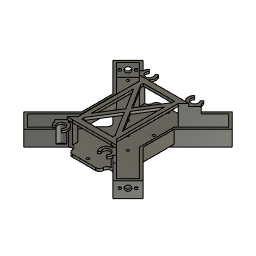
Frame_UAV2024 v2 (Autodesk Fusion 360 design; units mm, degrees)
Autodesk Fusion 360 part; units mm, degrees
sketch "スケッチ1" plane through (0, 0, 0) normal (0, 0, 1) x (1, 0, 0)
  line L0 (12, 34) -> (-12, 34)
  line L1 (-12, 34) -> (-12, -34)
  line L2 (-12, -34) -> (12, -34)
  line L3 (12, -34) -> (12, 34)
  line L4 (12, 34) -> (-12, -34) construction
  line L5 (-12, 34) -> (12, -34) construction
  line L6 (0, 0) -> (38.890873, 38.890873)
  line L7 (34.471456, 43.31029) -> (43.31029, 34.471456)
  line L8 (34.471456, 43.31029) -> (43.31029, 34.471456)
  line L9 (43.31029, 34.471456) -> (21.955666, 13.116831)
  line L10 (21.955666, 13.116831) -> (13.116831, 21.955666)
  line L11 (13.116831, 21.955666) -> (34.471456, 43.31029)
  line L12 (-34.471456, 43.31029) -> (-13.116831, 21.955666)
  line L13 (-13.116831, 21.955666) -> (-21.955666, 13.116831)
  line L14 (-21.955666, 13.116831) -> (-43.31029, 34.471456)
  line L15 (-43.31029, 34.471456) -> (-34.471456, 43.31029)
  line L16 (-43.31029, -34.471456) -> (-21.955666, -13.116831)
  line L17 (-21.955666, -13.116831) -> (-13.116831, -21.955666)
  line L18 (-13.116831, -21.955666) -> (-34.471456, -43.31029)
  line L19 (-34.471456, -43.31029) -> (-43.31029, -34.471456)
  line L20 (34.471456, -43.31029) -> (13.116831, -21.955666)
  line L21 (13.116831, -21.955666) -> (21.955666, -13.116831)
  line L22 (21.955666, -13.116831) -> (43.31029, -34.471456)
  line L23 (43.31029, -34.471456) -> (34.471456, -43.31029)
  line L24 (-10.288404, 21.955666) -> (-21.955666, 10.288404)
  line L25 (-21.955666, 10.288404) -> (-46.138717, 34.471456)
  line L26 (-46.138717, 34.471456) -> (-34.471456, 46.138717)
  line L27 (-34.471456, 46.138717) -> (-10.288404, 21.955666)
  line L28 (46.138717, 34.471456) -> (21.955666, 10.288404)
  line L29 (21.955666, 10.288404) -> (10.288404, 21.955666)
  line L30 (10.288404, 21.955666) -> (34.471456, 46.138717)
  line L31 (34.471456, 46.138717) -> (46.138717, 34.471456)
  line L32 (-46.138717, -34.471456) -> (-21.955666, -10.288404)
  line L33 (-21.955666, -10.288404) -> (-10.288404, -21.955666)
  line L34 (-10.288404, -21.955666) -> (-34.471456, -46.138717)
  line L35 (-34.471456, -46.138717) -> (-46.138717, -34.471456)
  line L36 (21.955666, -10.288404) -> (46.138717, -34.471456)
  line L37 (46.138717, -34.471456) -> (34.471456, -46.138717)
  line L38 (34.471456, -46.138717) -> (10.288404, -21.955666)
  line L39 (10.288404, -21.955666) -> (21.955666, -10.288404)
  line L40 (-10.288404, 21.955666) -> (-12, 23.667262)
  line L41 (10.288404, 21.955666) -> (12, 23.667262)
  line L42 (-10.288404, -21.955666) -> (-12, -23.667262)
  line L43 (10.288404, -21.955666) -> (12, -23.667262)
  line L44 (-21.955666, 10.288404) -> (-12, 0.332738)
  line L45 (-21.955666, 10.288404) -> (-6.411762, 10.288404) construction
  line L46 (-21.955666, -10.288404) -> (-12, -0.332738)
  line L47 (21.955666, 10.288404) -> (12, 0.332738)
  line L48 (21.955666, -10.288404) -> (12, -0.332738)
  dimension "d1" = 24
  dimension "d2" = 68
  dimension "d8" = 55
  dimension "d9" = 12.5
  dimension "d10" = 30.2
  dimension "d14" = 360
  dimension "d15" = -2
  dimension "d16" = -2
  dimension "d17" = -2
  dimension "d18" = -2
  dimension "d101" = 45
  dimension "d102" = 90
  dimension "d103" = 90
  constraint horizontal L0
  constraint perpendicular L0 L1
  constraint parallel L0 L2
  constraint parallel L1 L3
  constraint coincident L4 L6.start
  constraint coincident L5 L6.start
  constraint coincident L6.start origin
  constraint perpendicular L6 L7
  constraint perpendicular L8 L9
  constraint parallel L8 L10
  constraint parallel L9 L11
  constraint perpendicular L24 L40
  constraint perpendicular L29 L41
  constraint perpendicular L33 L42
  constraint perpendicular L39 L43
  constraint horizontal L45
  constraint perpendicular L24 L44
  constraint perpendicular L29 L47
  measures "d1" distance of L1.end L2.end
  measures "d2" distance of L0.end L1.end
  measures "d101" angle of L44 L45
  measures "d102" angle of L44 L46
  measures "d103" angle of L47 L48
extrude "押し出し1" add sketch "スケッチ1" along normal blind 2 contours L0 L1 L2 L3 L24 L27 L29 L30 L33 L34 L38 L39 L40 L41 L42 L43 | L3 L28 L29 L30 L31 | L3 L29 L30 L41 | L1 L24 L27 L40 | L1 L24 L25 L26 L27 | L3 L6 L29 | L1 L24 L44 | L3 L6 L29 L47 | L1 L33 L46 | L3 L39 L48 | L1 L33 L34 L42 | L1 L32 L33 L34 L35 | L3 L36 L37 L38 L39 | L3 L38 L39 L43 | L6 L7 L8 L10 L11 | L6 L7 L8 L9 L10 | L12 L13 L14 L15 | L16 L17 L18 L19 | L20 L21 L22 L23 picked at (3.429468, -7.540381) picked at (37.134891, 26.410438) picked at (11.429468, 21.955666) picked at (-11.429468, 21.955666) picked at (-30.016683, 19.29223) picked at (13.374012, 16.122035) picked at (-15.318555, 10.288404) picked at (15.318555, 7.540381) picked at (-15.318555, -10.288404) picked at (15.318555, -10.288404) picked at (-11.429468, -21.955666) picked at (-30.016683, -19.29223) picked at (30.016683, -19.29223) picked at (11.429468, -21.955666) picked at (28.826386, 34.718943) picked at (27.600735, 21.708178) picked at (-23.181317, 26.127596) picked at (-26.127596, -23.181317) picked at (23.181317, -26.127596)
sketch "スケッチ2" plane through (0, 0, 2) normal (0, 0, 1) x (-1, 0, 0)
  line L0 (12, 0.332738) -> (46.138717, 34.471456)
  line L1 (46.138717, 34.471456) -> (34.471456, 46.138717)
  line L2 (34.471456, 46.138717) -> (12, 23.667262)
  line L3 (12, 23.667262) -> (12, 34)
  line L4 (12, 34) -> (-12, 34)
  line L5 (-12, 34) -> (-12, 23.667262)
  line L6 (-12, 23.667262) -> (-34.471456, 46.138717)
  line L7 (-34.471456, 46.138717) -> (-46.138717, 34.471456)
  line L8 (-46.138717, 34.471456) -> (-12, 0.332738)
  line L9 (-12, 0.332738) -> (-12, -0.332738)
  line L10 (-12, -0.332738) -> (-46.138717, -34.471456)
  line L11 (-46.138717, -34.471456) -> (-34.471456, -46.138717)
  line L12 (-34.471456, -46.138717) -> (-12, -23.667262)
  line L13 (-12, -23.667262) -> (-12, -34)
  line L14 (-12, -34) -> (12, -34)
  line L15 (12, -34) -> (12, -23.667262)
  line L16 (12, -23.667262) -> (34.471456, -46.138717)
  line L17 (34.471456, -46.138717) -> (46.138717, -34.471456)
  line L18 (46.138717, -34.471456) -> (12, -0.332738)
  line L19 (12, -0.332738) -> (12, 0.332738)
  line L20 (-46.138717, -34.471456) -> (-34.471456, -46.138717)
  line L21 (-34.471456, -46.138717) -> (-12, -23.667262)
  line L22 (-12, -23.667262) -> (-23.667262, -12)
  line L23 (-23.667262, -12) -> (-46.138717, -34.471456)
  line L24 (-14.828427, -23.667262) -> (-23.667262, -14.828427)
  line L25 (-23.667262, -14.828427) -> (-43.31029, -34.471456)
  line L26 (-43.31029, -34.471456) -> (-34.471456, -43.31029)
  line L27 (-34.471456, -43.31029) -> (-14.828427, -23.667262)
  line L28 (-14.828427, -23.667262) -> (-13.414214, -22.253048)
  line L29 (-23.667262, -14.828427) -> (-22.253048, -13.414214)
  line L30 (-12, -23.667262) -> (-13.414214, -22.253048)
  line L31 (-22.253048, -13.414214) -> (-23.667262, -12)
  line L32 (43.31029, -34.471456) -> (23.667262, -14.828427)
  line L33 (34.471456, -43.31029) -> (43.31029, -34.471456)
  line L34 (14.828427, -23.667262) -> (34.471456, -43.31029)
  line L35 (14.828427, -23.667262) -> (13.414214, -22.253048)
  line L36 (23.667262, -14.828427) -> (22.253048, -13.414214)
  line L37 (23.667262, -12) -> (22.253048, -13.414214)
  line L38 (13.414214, -22.253048) -> (12, -23.667262)
  line L39 (34.471456, 43.31029) -> (14.828427, 23.667262)
  line L40 (43.31029, 34.471456) -> (34.471456, 43.31029)
  line L41 (23.667262, 14.828427) -> (43.31029, 34.471456)
  line L42 (23.667262, 14.828427) -> (22.253048, 13.414214)
  line L43 (14.828427, 23.667262) -> (13.414214, 22.253048)
  line L44 (12, 23.667262) -> (13.414214, 22.253048)
  line L45 (22.253048, 13.414214) -> (23.667262, 12)
  line L46 (-43.31029, 34.471456) -> (-23.667262, 14.828427)
  line L47 (-34.471456, 43.31029) -> (-43.31029, 34.471456)
  line L48 (-14.828427, 23.667262) -> (-34.471456, 43.31029)
  line L49 (-14.828427, 23.667262) -> (-13.414214, 22.253048)
  line L50 (-23.667262, 14.828427) -> (-22.253048, 13.414214)
  line L51 (-23.667262, 12) -> (-22.253048, 13.414214)
  line L52 (-13.414214, 22.253048) -> (-12, 23.667262)
  dimension "d105" = -2
  dimension "d107" = 360
  constraint perpendicular L20 L21
  constraint parallel L20 L22
  constraint parallel L21 L23
  constraint perpendicular L12 L20
  constraint perpendicular L22 L28
  constraint perpendicular L22 L29
  constraint perpendicular L28 L30
extrude "押し出し2" add sketch "スケッチ2" along normal blind 10 contours L0 L1 L2 L39 L40 L41 L42 L43 L44 L45 | L16 L17 L18 L32 L33 L34 L35 L36 L37 L38 | L6 L7 L8 L46 L47 L48 L49 L50 L51 L52 | L10 L11 L12 L20 L21 L22 L23 L25 L26 L27 L28 L29 L30 L31 picked at (31.157747, 20.433294) picked at (20.433294, -31.157747) picked at (-20.433294, 31.157747) picked at (-31.157747, -20.433294)
sketch "スケッチ3" plane through (-40.305087, 40.305087, 0) normal (-0.707107, 0.707107, 0) x (-0.707107, -0.707107, 0)
  line L0 (-8.25, 0) -> (8.25, 0)
  line L1 (8.25, 0) -> (8.25, 12)
  line L2 (8.25, 12) -> (-8.25, 12)
  line L3 (-8.25, 12) -> (-8.25, 0)
  line L4 (0, 12) -> (0, 7)
  circle A0 centre (0, 7) radius 2.1
  line L5 (0, 7) -> (4.5, 7)
  circle A1 centre (4.5, 7) radius 1
  line L6 (0, 7) -> (-4.5, 7)
  circle A2 centre (-4.5, 7) radius 1
  dimension "d33" = 4.2
  dimension "d34" = 4.5
  dimension "d35" = 2
  dimension "d36" = 4.5
  dimension "d37" = 2
  constraint midpoint L2 L4.start
  constraint perpendicular L2 L4
  constraint coincident L4.end A0.centre
  constraint perpendicular L4 L5
  constraint coincident L5.end A1.centre
  constraint perpendicular L4 L6
  constraint coincident L6.end A2.centre
  measures "d33" diameter of A0
  measures "d34" distance of L4.end L5.end
  measures "d35" diameter of A1
  measures "d36" distance of L4.end L6.end
  measures "d37" diameter of A2
extrude "押し出し3" cut sketch "スケッチ3" against normal blind 2 contours L4 A0 L5 | L4 A0 L6 | A0 L5 L6 | A1 | A2 picked at (1.308387, 7.488003) picked at (-1.117902, 7.836851) picked at (-1.392182, 6.895671) picked at (4.70783, 6.807162) picked at (-4.121993, 6.641138)
pattern_circular "C パターン1" count 4 over 360 about axis through (0, 0, 1.75) along (0, 0, 1) of "押し出し3"
ref_plane "作業平面4" through (0, 0, 12) normal (0, 0, 1) x (1, 0, 0)
sketch "スケッチ24" plane through (0, 0, 12) normal (0, 0, 1) x (1, 0, 0)
  line L0 (17.5, 34) -> (-17.5, 34)
  line L1 (-17.5, 34) -> (-17.5, -34)
  line L2 (-17.5, -34) -> (17.5, -34)
  line L3 (17.5, -34) -> (17.5, 34)
  line L4 (17.5, 34) -> (-17.5, -34) construction
  line L5 (-17.5, 34) -> (17.5, -34) construction
  circle A0 centre (-17.5, 34) radius 3
  line L6 (-46.138717, -34.471456) -> (-12, -0.332738)
  line L7 (-12, -0.332738) -> (-12, 0.332738)
  line L8 (-12, 0.332738) -> (-46.138717, 34.471456)
  line L9 (-46.138717, 34.471456) -> (-34.471456, 46.138717)
  line L10 (-34.471456, 46.138717) -> (-12, 23.667262)
  line L11 (-12, 23.667262) -> (-12, 34)
  line L12 (-12, 34) -> (12, 34)
  line L13 (12, 34) -> (12, 23.667262)
  line L14 (12, 23.667262) -> (34.471456, 46.138717)
  line L15 (34.471456, 46.138717) -> (46.138717, 34.471456)
  line L16 (46.138717, 34.471456) -> (12, 0.332738)
  line L17 (12, 0.332738) -> (12, -0.332738)
  line L18 (12, -0.332738) -> (46.138717, -34.471456)
  line L19 (46.138717, -34.471456) -> (34.471456, -46.138717)
  line L20 (34.471456, -46.138717) -> (12, -23.667262)
  line L21 (12, -23.667262) -> (12, -34)
  line L22 (12, -34) -> (-12, -34)
  line L23 (-12, -34) -> (-12, -23.667262)
  line L24 (-12, -23.667262) -> (-34.471456, -46.138717)
  line L25 (-34.471456, -46.138717) -> (-46.138717, -34.471456)
  circle A1 centre (17.5, 34) radius 3
  circle A2 centre (-17.5, -34) radius 3
  circle A3 centre (17.5, -34) radius 3
  circle A4 centre (-17.5, 34) radius 5
  circle A5 centre (17.5, 34) radius 5
  circle A6 centre (-17.5, -34) radius 5
  circle A7 centre (17.5, -34) radius 5
  dimension "d119" = 35
  dimension "d120" = 68
  dimension "d122" = 6
  dimension "d125" = 6
  dimension "d126" = 6
  dimension "d127" = 6
  dimension "d152" = 10
  dimension "d153" = 10
  dimension "d154" = 10
  dimension "d155" = 10
  constraint horizontal L0
  constraint perpendicular L0 L1
  constraint parallel L0 L2
  constraint parallel L1 L3
  constraint coincident L4 origin
  constraint coincident L5 origin
  constraint coincident L0.end L1.start
  constraint coincident L0.start L3.end
  constraint coincident L1.end L2.start
  constraint coincident L2.end L3.start
  constraint concentric A0 A4
  constraint concentric A1 A5
  constraint concentric A2 A6
  constraint concentric A3 A7
  measures "d119" distance of L1.end L2.end
  measures "d120" distance of L0.end L1.end
  measures "d122" diameter of A0
  measures "d125" diameter of A1
  measures "d126" diameter of A2
  measures "d127" diameter of A3
  measures "d152" diameter of A4
  measures "d153" diameter of A5
  measures "d154" diameter of A6
  measures "d155" diameter of A7
extrude "押し出し22" add sketch "スケッチ24" against normal blind 1.5 contours L0 L3 L14 A1 A5 | L0 L3 L14 A1 A5 | L0 L1 A0 L10 A4 | L0 L1 A0 L10 A4 | L2 L3 L20 A3 A7 | L2 L3 L20 A3 A7 | L1 L2 L24 A2 A6 | L1 L2 L24 A2 A6 picked at (21.79405, 34.503832) picked at (17.071241, 29.757399) picked at (-17.071241, 29.757399) picked at (-21.804015, 34.403857) picked at (21.79405, -34.503832) picked at (17.071241, -29.757399) picked at (-17.071241, -29.757399) picked at (-21.804015, -34.403857)
sketch "スケッチ25" plane through (0, 0, 2) normal (0, 0, 1) x (-1, 0, 0)
  line L0 (22.253048, -13.414214) -> (23.667262, -12)
  line L1 (23.667262, -12) -> (12, -0.332738)
  line L2 (12, -0.332738) -> (12, 0.332738)
  line L3 (12, 0.332738) -> (23.667262, 12)
  line L4 (23.667262, 12) -> (22.253048, 13.414214)
  line L5 (22.253048, 13.414214) -> (43.31029, 34.471456)
  line L6 (43.31029, 34.471456) -> (34.471456, 43.31029)
  line L7 (34.471456, 43.31029) -> (13.414214, 22.253048)
  line L8 (13.414214, 22.253048) -> (12, 23.667262)
  line L9 (12, 23.667262) -> (12, 34)
  line L10 (12, 34) -> (-12, 34)
  line L11 (-12, 34) -> (-12, 23.667262)
  line L12 (-12, 23.667262) -> (-13.414214, 22.253048)
  line L13 (-13.414214, 22.253048) -> (-34.471456, 43.31029)
  line L14 (-34.471456, 43.31029) -> (-43.31029, 34.471456)
  line L15 (-43.31029, 34.471456) -> (-22.253048, 13.414214)
  line L16 (-22.253048, 13.414214) -> (-23.667262, 12)
  line L17 (-23.667262, 12) -> (-12, 0.332738)
  line L18 (-12, 0.332738) -> (-12, -0.332738)
  line L19 (-12, -0.332738) -> (-23.667262, -12)
  line L20 (-23.667262, -12) -> (-22.253048, -13.414214)
  line L21 (-22.253048, -13.414214) -> (-43.31029, -34.471456)
  line L22 (-43.31029, -34.471456) -> (-34.471456, -43.31029)
  line L23 (-34.471456, -43.31029) -> (-13.414214, -22.253048)
  line L24 (-13.414214, -22.253048) -> (-12, -23.667262)
  line L25 (-12, -23.667262) -> (-12, -34)
  line L26 (-12, -34) -> (12, -34)
  line L27 (12, -34) -> (12, -23.667262)
  line L28 (12, -23.667262) -> (13.414214, -22.253048)
  line L29 (13.414214, -22.253048) -> (34.471456, -43.31029)
  line L30 (34.471456, -43.31029) -> (43.31029, -34.471456)
  line L31 (43.31029, -34.471456) -> (22.253048, -13.414214)
  line L32 (17.5, -34) -> (-17.5, -34)
  line L33 (-17.5, -34) -> (-17.5, 34)
  line L34 (-17.5, 34) -> (17.5, 34)
  line L35 (17.5, 34) -> (17.5, -34)
  line L36 (17.5, -34) -> (-17.5, 34) construction
  line L37 (-17.5, -34) -> (17.5, 34) construction
  circle A0 centre (17.5, -34) radius 4.5
  circle A1 centre (-17.5, -34) radius 4.5
  circle A2 centre (17.5, 34) radius 4.5
  circle A3 centre (-17.5, 34) radius 4.5
  dimension "d130" = 35
  dimension "d131" = 68
  dimension "d132" = 9
  dimension "d133" = 9
  dimension "d134" = 9
  dimension "d135" = 9
  constraint horizontal L32
  constraint perpendicular L32 L33
  constraint parallel L32 L34
  constraint parallel L33 L35
  constraint coincident L36 origin
  constraint coincident L37 origin
  constraint coincident L32.start L35.end
  constraint coincident L32.end L33.start
  constraint coincident L34.end L35.start
  constraint coincident L33.end L34.start
  measures "d130" distance of L33.end L34.end
  measures "d131" distance of L32.end L33.end
  measures "d132" diameter of A0
  measures "d133" diameter of A1
  measures "d134" diameter of A2
  measures "d135" diameter of A3
extrude "押し出し23" cut sketch "スケッチ25" along normal blind 8.5 contours L32 L35 A0 | L32 L35 A0 | L34 L35 A2 | L34 L35 A2 | L32 L33 A1 | L32 L33 A1 | L33 L34 A3 | L33 L34 A3 picked at (14.516754, -34.223563) picked at (14.873672, -32.565916) picked at (14.515268, 33.786528) picked at (14.583395, 34.665696) picked at (-14.580825, -34.655523) picked at (-14.576028, -33.363929) picked at (-14.515268, 33.786528) picked at (-18.57676, 31.208606)
sketch "スケッチ26" plane through (0, 0, 12) normal (0, 0, 1) x (1, 0, 0)
  circle A0 centre (-17.5, 34) radius 3
  circle A1 centre (17.5, 34) radius 3
  circle A2 centre (-17.5, -34) radius 3
  circle A3 centre (17.5, -34) radius 3
  line L0 (-17.5, 34) -> (-13.610913, 37.889087)
  line L1 (-17.5, 34) -> (-12, 34) construction
  arc A4 (-13.610913, 37.889087) -> (-21.389087, 37.889087) centre (-17.5, 34) ccw
  line L2 (-17.5, 34) -> (-21.389087, 37.889087)
  line L3 (0, 2.5) -> (0, 20)
  line L4 (17.5, 34) -> (21.389087, 37.889087)
  line L5 (17.5, 34) -> (13.610913, 37.889087)
  arc A5 (21.389087, 37.889087) -> (13.610913, 37.889087) centre (17.5, 34) ccw
  line L6 (20, 0) -> (2.5, 0)
  line L7 (-17.5, -34) -> (-13.610913, -37.889087)
  line L8 (-17.5, -34) -> (-21.389087, -37.889087)
  arc A6 (-21.389087, -37.889087) -> (-13.610913, -37.889087) centre (-17.5, -34) ccw
  line L9 (17.5, -34) -> (21.389087, -37.889087)
  line L10 (17.5, -34) -> (13.610913, -37.889087)
  arc A7 (13.610913, -37.889087) -> (21.389087, -37.889087) centre (17.5, -34) ccw
  dimension "d138" = 45
  constraint horizontal L1
  constraint coincident A0.centre L0.start
  constraint symmetric A0.centre L3 A1.centre
  constraint symmetric A4 L3 A5
  constraint symmetric A0.centre L6 A2.centre
  constraint symmetric A4 L6 A6
  constraint symmetric A1.centre L6 A3.centre
  constraint symmetric A5 L6 A7
  measures "d138" angle of L0 L1
extrude "押し出し24" cut sketch "スケッチ26" against normal blind 1.5 contours A0 L0 A4 L2 | A1 L4 L5 A5 | A2 L7 L8 A6 | A3 L9 L10 A7 picked at (-15.043452, 37.954416) picked at (19.956548, 37.954416) picked at (-15.043452, -37.954416) picked at (19.368772, -38.263769)
sketch "スケッチ27" plane through (0, 0, 0) normal (0, 0, -1) x (1, 0, 0)
  line L0 (-46.138717, 34.471456) -> (-12, 0.332738)
  line L1 (-12, 0.332738) -> (-12, -0.332738)
  line L2 (-12, -0.332738) -> (-46.138717, -34.471456)
  line L3 (-46.138717, -34.471456) -> (-34.471456, -46.138717)
  line L4 (-34.471456, -46.138717) -> (-12, -23.667262)
  line L5 (-12, -23.667262) -> (-12, -34)
  line L6 (-12, -34) -> (12, -34)
  line L7 (12, -34) -> (12, -23.667262)
  line L8 (12, -23.667262) -> (34.471456, -46.138717)
  line L9 (34.471456, -46.138717) -> (46.138717, -34.471456)
  line L10 (46.138717, -34.471456) -> (12, -0.332738)
  line L11 (12, -0.332738) -> (12, 0.332738)
  line L12 (12, 0.332738) -> (46.138717, 34.471456)
  line L13 (46.138717, 34.471456) -> (34.471456, 46.138717)
  line L14 (34.471456, 46.138717) -> (12, 23.667262)
  line L15 (12, 23.667262) -> (12, 34)
  line L16 (12, 34) -> (-12, 34)
  line L17 (-12, 34) -> (-12, 23.667262)
  line L18 (-12, 23.667262) -> (-34.471456, 46.138717)
  line L19 (-34.471456, 46.138717) -> (-46.138717, 34.471456)
  line L20 (10, -10) -> (-10, -10)
  line L21 (-10, -10) -> (-10, 10)
  line L22 (-10, 10) -> (10, 10)
  line L23 (10, 10) -> (10, -10)
  line L24 (10, -10) -> (-10, 10) construction
  line L25 (-10, -10) -> (10, 10) construction
  circle A0 centre (-10, 10) radius 0.9
  circle A1 centre (-10, 10) radius 2.5
  circle A2 centre (-10, -10) radius 2.5
  circle A3 centre (-10, -10) radius 0.9
  circle A4 centre (10, -10) radius 2.5
  circle A5 centre (10, -10) radius 0.9
  circle A6 centre (10, 10) radius 2.5
  circle A7 centre (10, 10) radius 0.9
  dimension "d141" = 20
  dimension "d142" = 20
  dimension "d143" = 1.8
  dimension "d144" = 5
  dimension "d146" = 360
  constraint horizontal L20
  constraint perpendicular L20 L21
  constraint parallel L20 L22
  constraint parallel L21 L23
  constraint coincident L24 origin
  constraint coincident L25 origin
  constraint coincident L21.end L22.start
  measures "d141" distance of L21.end L22.end
  measures "d142" distance of L20.end L21.end
  measures "d143" diameter of A0
  measures "d144" diameter of A1
extrude "押し出し25" add sketch "スケッチ27" along normal blind 5 contours L20 L21 A2 A3 | L20 L21 A2 A3 | L20 L23 A4 A5 | L20 L23 A4 A5 | L21 L22 A0 A1 | L21 L22 A0 A1 | L22 L23 A6 A7 | L22 L23 A6 A7 picked at (-9.929804, -11.960206) picked at (-8.628033, -8.597767) picked at (8.044869, -9.83871) picked at (11.957359, -10.124202) picked at (-10.122275, 8.042353) picked at (-9.881404, 8.041815) picked at (8.078625, 9.603933) picked at (8.045992, 10.168915)
sketch "スケッチ28" plane through (0, 0, 12) normal (0, 0, 1) x (1, 0, 0)
  line L0 (-12, 34.000001) -> (12, 34.000001)
  line L1 (12, 34.000001) -> (12, -34.000001)
  line L2 (12, -34.000001) -> (-12, -34.000001)
  line L3 (-12, -34.000001) -> (-12, 34.000001)
  line L4 (-12, 34.000001) -> (12, -34.000001) construction
  line L5 (12, 34.000001) -> (-12, -34.000001) construction
  line L6 (15, 37.000001) -> (15, -37.000001)
  line L7 (15, -37.000001) -> (-15, -37.000001)
  line L8 (-15, -37.000001) -> (-15, 37.000001)
  line L9 (-15, 37.000001) -> (15, 37.000001)
  line L10 (-13.964466, 37.535534) -> (-15.37868, 36.12132)
  arc A0 (-15.37868, 36.12132) -> (-19.62132, 36.12132) centre (-17.5, 34) cw
  line L11 (-19.62132, 36.12132) -> (-21.035534, 37.535534)
  arc A1 (-21.035534, 37.535534) -> (-22.497291, 34.164553) centre (-17.5, 34) ccw
  line L12 (-22.497291, 34.164553) -> (-34.471456, 46.138717)
  line L13 (-34.471456, 46.138717) -> (-46.138717, 34.471456)
  line L14 (-46.138717, 34.471456) -> (-23.667262, 12)
  line L15 (-23.667262, 12) -> (-22.253048, 13.414214)
  line L16 (-22.253048, 13.414214) -> (-43.31029, 34.471456)
  line L17 (-43.31029, 34.471456) -> (-34.471456, 43.31029)
  line L18 (-34.471456, 43.31029) -> (-13.414214, 22.253048)
  line L19 (-13.414214, 22.253048) -> (-12, 23.667262)
  line L20 (-12, 23.667262) -> (-17.335447, 29.002709)
  arc A2 (-17.335447, 29.002709) -> (-13.964466, 37.535534) centre (-17.5, 34) ccw
  line L21 (21.035534, 37.535534) -> (19.62132, 36.12132)
  arc A3 (19.62132, 36.12132) -> (15.37868, 36.12132) centre (17.5, 34) cw
  line L22 (15.37868, 36.12132) -> (13.964466, 37.535534)
  arc A4 (13.964466, 37.535534) -> (17.335447, 29.002709) centre (17.5, 34) ccw
  line L23 (17.335447, 29.002709) -> (12, 23.667262)
  line L24 (12, 23.667262) -> (13.414214, 22.253048)
  line L25 (13.414214, 22.253048) -> (34.471456, 43.31029)
  line L26 (34.471456, 43.31029) -> (43.31029, 34.471456)
  line L27 (43.31029, 34.471456) -> (22.253048, 13.414214)
  line L28 (22.253048, 13.414214) -> (23.667262, 12)
  line L29 (23.667262, 12) -> (46.138717, 34.471456)
  line L30 (46.138717, 34.471456) -> (34.471456, 46.138717)
  line L31 (34.471456, 46.138717) -> (22.497291, 34.164553)
  arc A5 (22.497291, 34.164553) -> (21.035534, 37.535534) centre (17.5, 34) ccw
  line L32 (-21.035534, -37.535534) -> (-19.62132, -36.12132)
  arc A6 (-19.62132, -36.12132) -> (-15.37868, -36.12132) centre (-17.5, -34) cw
  line L33 (-15.37868, -36.12132) -> (-13.964466, -37.535534)
  arc A7 (-13.964466, -37.535534) -> (-17.335447, -29.002709) centre (-17.5, -34) ccw
  line L34 (-17.335447, -29.002709) -> (-12, -23.667262)
  line L35 (-12, -23.667262) -> (-13.414214, -22.253048)
  line L36 (-13.414214, -22.253048) -> (-34.471456, -43.31029)
  line L37 (-34.471456, -43.31029) -> (-43.31029, -34.471456)
  line L38 (-43.31029, -34.471456) -> (-22.253048, -13.414214)
  line L39 (-22.253048, -13.414214) -> (-23.667262, -12)
  line L40 (-23.667262, -12) -> (-46.138717, -34.471456)
  line L41 (-46.138717, -34.471456) -> (-34.471456, -46.138717)
  line L42 (-34.471456, -46.138717) -> (-22.497291, -34.164553)
  arc A8 (-22.497291, -34.164553) -> (-21.035534, -37.535534) centre (-17.5, -34) ccw
  line L43 (13.964466, -37.535534) -> (15.37868, -36.12132)
  arc A9 (15.37868, -36.12132) -> (19.62132, -36.12132) centre (17.5, -34) cw
  line L44 (19.62132, -36.12132) -> (21.035534, -37.535534)
  arc A10 (21.035534, -37.535534) -> (22.497291, -34.164553) centre (17.5, -34) ccw
  line L45 (22.497291, -34.164553) -> (34.471456, -46.138717)
  line L46 (34.471456, -46.138717) -> (46.138717, -34.471456)
  line L47 (46.138717, -34.471456) -> (23.667262, -12)
  line L48 (23.667262, -12) -> (22.253048, -13.414214)
  line L49 (22.253048, -13.414214) -> (43.31029, -34.471456)
  line L50 (43.31029, -34.471456) -> (34.471456, -43.31029)
  line L51 (34.471456, -43.31029) -> (13.414214, -22.253048)
  line L52 (13.414214, -22.253048) -> (12, -23.667262)
  line L53 (12, -23.667262) -> (17.335447, -29.002709)
  arc A11 (17.335447, -29.002709) -> (13.964466, -37.535534) centre (17.5, -34) ccw
  dimension "d149" = -3
  constraint horizontal L0
  constraint perpendicular L0 L1
  constraint parallel L0 L2
  constraint parallel L1 L3
  constraint coincident L4 origin
  constraint coincident L5 origin
extrude "押し出し26" cut sketch "スケッチ28" against normal blind 10 contours L8 L18 L19 L20 | L6 L23 L24 L25 | L8 L34 L35 L36 | L6 L51 L52 L53 picked at (-14, 24.724453) picked at (14, 24.724453) picked at (-14, -24.724453) picked at (14, -24.724453)
extrude "押し出し27" cut 4 faces at (9.731307, 10.009657, 0) (-10.083244, 10.032671, 0) (-10.182869, -9.709695, 0) (10.356587, -10.144182, 0) along direction (0, 0, 1) blind 2
fillet "フィレット1" radius 3 8 edges at (12, 23.667262, 1) (-12, 23.667262, 1) (12, -23.667262, 1) (-12, -23.667262, 1) (-12, 0.332738, 1) (-12, -0.332738, 1) (12, -0.332738, 1) (12, 0.332738, 1)
fillet "フィレット2" radius 3 4 edges at (12, 34, 1) (-12, 34, 1) (-12, -34, 1) (12, -34, 1)
sketch "スケッチ29" plane through (0, 0, 2) normal (0, 0, 1) x (-1, 0, 0)
  arc A0 (-9, 34) -> (-12, 31) centre (-9, 31) ccw
  line L0 (-12, 31) -> (-12, 30.909903)
  arc A1 (-15, 27.909903) -> (-12, 30.909903) centre (-15, 30.909903) ccw
  line L1 (-15, 27.909903) -> (-15, 23.838835)
  line L2 (-15, 23.838835) -> (-34.471456, 43.31029)
  line L3 (-34.471456, 43.31029) -> (-43.31029, 34.471456)
  line L4 (-43.31029, 34.471456) -> (-22.253048, 13.414214)
  line L5 (-22.253048, 13.414214) -> (-23.667262, 12)
  line L6 (-23.667262, 12) -> (-13.788582, 2.12132)
  arc A2 (-13.788582, -2.12132) -> (-13.788582, 2.12132) centre (-15.909903, 0) ccw
  line L7 (-13.788582, -2.12132) -> (-23.667262, -12)
  line L8 (-23.667262, -12) -> (-22.253048, -13.414214)
  line L9 (-22.253048, -13.414214) -> (-43.31029, -34.471456)
  line L10 (-43.31029, -34.471456) -> (-34.471456, -43.31029)
  line L11 (-34.471456, -43.31029) -> (-15, -23.838835)
  line L12 (-15, -23.838835) -> (-15, -27.909903)
  arc A3 (-12, -30.909903) -> (-15, -27.909903) centre (-15, -30.909903) ccw
  line L13 (-12, -30.909903) -> (-12, -31)
  arc A4 (-12, -31) -> (-9, -34) centre (-9, -31) ccw
  line L14 (-9, -34) -> (9, -34)
  arc A5 (9, -34) -> (12, -31) centre (9, -31) ccw
  line L15 (12, -31) -> (12, -30.909903)
  arc A6 (15, -27.909903) -> (12, -30.909903) centre (15, -30.909903) ccw
  line L16 (15, -27.909903) -> (15, -23.838835)
  line L17 (15, -23.838835) -> (34.471456, -43.31029)
  line L18 (34.471456, -43.31029) -> (43.31029, -34.471456)
  line L19 (43.31029, -34.471456) -> (22.253048, -13.414214)
  line L20 (22.253048, -13.414214) -> (23.667262, -12)
  line L21 (23.667262, -12) -> (13.788582, -2.12132)
  line L22 (13.788582, 2.12132) -> (23.667262, 12)
  line L23 (23.667262, 12) -> (22.253048, 13.414214)
  line L24 (22.253048, 13.414214) -> (43.31029, 34.471456)
  line L25 (43.31029, 34.471456) -> (34.471456, 43.31029)
  line L26 (34.471456, 43.31029) -> (15, 23.838835)
  line L27 (15, 23.838835) -> (15, 27.909903)
  arc A7 (12, 30.909903) -> (15, 27.909903) centre (15, 30.909903) ccw
  line L28 (12, 30.909903) -> (12, 31)
  arc A8 (12, 31) -> (9, 34) centre (9, 31) ccw
  line L29 (9, 34) -> (-9, 34)
  circle A9 centre (10, 10) radius 0.9
  circle A10 centre (-10, -10) radius 0.9
  circle A11 centre (10, -10) radius 0.9
  circle A12 centre (-10, 10) radius 0.9
  line L30 (23.667262, -12) -> (23.667262, 12)
  line L31 (22.253048, -13.414214) -> (22.253048, 13.414214)
  line L32 (-23.667262, -12) -> (-23.667262, 12)
  line L33 (-22.253048, -13.414214) -> (-22.253048, 13.414214)
  arc A13 (13.788582, 2.12132) -> (13.788582, -2.12132) centre (15.909903, 0) ccw
extrude "押し出し28" add sketch "スケッチ29" along normal blind 10 contours L5 L6 L33 | L6 L7 L32 L33 | L22 L23 L31 | L7 L8 L33 | L21 L22 L30 L31 | L20 L21 L31 picked at (-22.724453, 12) picked at (-23.195857, 3.528595) picked at (22.724453, 12) picked at (-22.724453, -12) picked at (23.195857, 3.528595) picked at (22.724453, -12)
sketch "スケッチ30" plane through (0, 0, 12) normal (0, 0, 1) x (-1, 0, 0)
  line L0 (15, -23.838835) -> (15, -27.909903)
  arc A0 (17.12132, -28.788582) -> (15, -27.909903) centre (15, -30.909903) ccw
  line L1 (17.12132, -28.788582) -> (17.335447, -29.002709)
  arc A1 (17.335447, -29.002709) -> (13.964466, -37.535534) centre (17.5, -34) ccw
  line L2 (13.964466, -37.535534) -> (15.37868, -36.12132)
  arc A2 (19.62132, -36.12132) -> (15.37868, -36.12132) centre (17.5, -34) ccw
  line L3 (19.62132, -36.12132) -> (21.035534, -37.535534)
  arc A3 (21.035534, -37.535534) -> (22.497291, -34.164553) centre (17.5, -34) ccw
  line L4 (22.497291, -34.164553) -> (34.471456, -46.138717)
  line L5 (34.471456, -46.138717) -> (46.138717, -34.471456)
  line L6 (46.138717, -34.471456) -> (23.667262, -12)
  line L7 (23.667262, -12) -> (23.667262, 12)
  line L8 (23.667262, 12) -> (46.138717, 34.471456)
  line L9 (46.138717, 34.471456) -> (34.471456, 46.138717)
  line L10 (34.471456, 46.138717) -> (22.497291, 34.164553)
  arc A4 (22.497291, 34.164553) -> (21.035534, 37.535534) centre (17.5, 34) ccw
  line L11 (21.035534, 37.535534) -> (19.62132, 36.12132)
  arc A5 (15.37868, 36.12132) -> (19.62132, 36.12132) centre (17.5, 34) ccw
  line L12 (15.37868, 36.12132) -> (13.964466, 37.535534)
  arc A6 (13.964466, 37.535534) -> (17.335447, 29.002709) centre (17.5, 34) ccw
  line L13 (17.335447, 29.002709) -> (17.12132, 28.788582)
  arc A7 (15, 27.909903) -> (17.12132, 28.788582) centre (15, 30.909903) ccw
  line L14 (15, 27.909903) -> (15, 23.838835)
  line L15 (15, 23.838835) -> (34.471456, 43.31029)
  line L16 (34.471456, 43.31029) -> (43.31029, 34.471456)
  line L17 (43.31029, 34.471456) -> (22.253048, 13.414214)
  line L18 (22.253048, 13.414214) -> (22.253048, -13.414214)
  line L19 (22.253048, -13.414214) -> (43.31029, -34.471456)
  line L20 (43.31029, -34.471456) -> (34.471456, -43.31029)
  line L21 (34.471456, -43.31029) -> (15, -23.838835)
  line L22 (-15, 23.838835) -> (-15, 27.909903)
  arc A8 (-17.12132, 28.788582) -> (-15, 27.909903) centre (-15, 30.909903) ccw
  line L23 (-17.12132, 28.788582) -> (-17.335447, 29.002709)
  arc A9 (-17.335447, 29.002709) -> (-13.964466, 37.535534) centre (-17.5, 34) ccw
  line L24 (-13.964466, 37.535534) -> (-15.37868, 36.12132)
  arc A10 (-19.62132, 36.12132) -> (-15.37868, 36.12132) centre (-17.5, 34) ccw
  line L25 (-19.62132, 36.12132) -> (-21.035534, 37.535534)
  arc A11 (-21.035534, 37.535534) -> (-22.497291, 34.164553) centre (-17.5, 34) ccw
  line L26 (-22.497291, 34.164553) -> (-34.471456, 46.138717)
  line L27 (-34.471456, 46.138717) -> (-46.138717, 34.471456)
  line L28 (-46.138717, 34.471456) -> (-23.667262, 12)
  line L29 (-23.667262, 12) -> (-23.667262, -12)
  line L30 (-23.667262, -12) -> (-46.138717, -34.471456)
  line L31 (-46.138717, -34.471456) -> (-34.471456, -46.138717)
  line L32 (-34.471456, -46.138717) -> (-22.497291, -34.164553)
  arc A12 (-22.497291, -34.164553) -> (-21.035534, -37.535534) centre (-17.5, -34) ccw
  line L33 (-21.035534, -37.535534) -> (-19.62132, -36.12132)
  arc A13 (-15.37868, -36.12132) -> (-19.62132, -36.12132) centre (-17.5, -34) ccw
  line L34 (-15.37868, -36.12132) -> (-13.964466, -37.535534)
  arc A14 (-13.964466, -37.535534) -> (-17.335447, -29.002709) centre (-17.5, -34) ccw
  line L35 (-17.335447, -29.002709) -> (-17.12132, -28.788582)
  arc A15 (-15, -27.909903) -> (-17.12132, -28.788582) centre (-15, -30.909903) ccw
  line L36 (-15, -27.909903) -> (-15, -23.838835)
  line L37 (-15, -23.838835) -> (-34.471456, -43.31029)
  line L38 (-34.471456, -43.31029) -> (-43.31029, -34.471456)
  line L39 (-43.31029, -34.471456) -> (-22.253048, -13.414214)
  line L40 (-22.253048, -13.414214) -> (-22.253048, 13.414214)
  line L41 (-22.253048, 13.414214) -> (-43.31029, 34.471456)
  line L42 (-43.31029, 34.471456) -> (-34.471456, 43.31029)
  line L43 (-34.471456, 43.31029) -> (-15, 23.838835)
  circle A16 centre (17.5, 34) radius 5
  circle A17 centre (17.5, -34) radius 5
  circle A18 centre (-17.5, -34) radius 5
  circle A19 centre (-17.5, 34) radius 5
  constraint concentric A4 A16
  constraint concentric A1 A17
  constraint concentric A12 A18
  constraint concentric A9 A19
extrude "押し出し29" add sketch "スケッチ30" along normal blind 5 contours A1 L2 A2 L3 A3 A17 | A4 L11 A5 L12 A6 A16 | A9 L24 A10 L25 A11 A19 | A12 L33 A13 L34 A14 A18 picked at (21.810837, -33.659856) picked at (21.810837, 33.659856) picked at (-17.63783, 29.678745) picked at (-17.63783, -29.678745)
extrude "押し出し30" cut 4 faces at (-17.173323, -29.874969, 10.5) (17.173323, -29.874969, 10.5) (17.173323, 29.874969, 10.5) (-17.173323, 29.874969, 10.5) along direction (0, 0, 1) blind 5
sketch "スケッチ31" plane through (0, 0, 2) normal (0, 0, 1) x (-1, 0, 0)
  line L0 (-22.253048, 13.414214) -> (-22.253048, 10.585786)
  line L1 (-22.253048, 10.585786) -> (-13.788582, 2.12132)
  arc A0 (-13.788582, -2.12132) -> (-13.788582, 2.12132) centre (-15.909903, 0) ccw
  line L2 (-13.788582, -2.12132) -> (-22.253048, -10.585786)
  line L3 (-22.253048, -10.585786) -> (-22.253048, -13.414214)
  line L4 (-22.253048, -13.414214) -> (-43.31029, -34.471456)
  line L5 (-43.31029, -34.471456) -> (-34.471456, -43.31029)
  line L6 (-34.471456, -43.31029) -> (-15, -23.838835)
  line L7 (-15, -23.838835) -> (-15, -27.909903)
  arc A1 (-12, -30.909903) -> (-15, -27.909903) centre (-15, -30.909903) ccw
  line L8 (-12, -30.909903) -> (-12, -31)
  arc A2 (-12, -31) -> (-9, -34) centre (-9, -31) ccw
  line L9 (-9, -34) -> (9, -34)
  arc A3 (9, -34) -> (12, -31) centre (9, -31) ccw
  line L10 (12, -31) -> (12, -30.909903)
  arc A4 (15, -27.909903) -> (12, -30.909903) centre (15, -30.909903) ccw
  line L11 (15, -27.909903) -> (15, -23.838835)
  line L12 (15, -23.838835) -> (34.471456, -43.31029)
  line L13 (34.471456, -43.31029) -> (43.31029, -34.471456)
  line L14 (43.31029, -34.471456) -> (22.253048, -13.414214)
  line L15 (22.253048, -13.414214) -> (22.253048, -10.585786)
  line L16 (22.253048, -10.585786) -> (13.788582, -2.12132)
  line L17 (13.788582, 2.12132) -> (22.253048, 10.585786)
  line L18 (22.253048, 10.585786) -> (22.253048, 13.414214)
  line L19 (22.253048, 13.414214) -> (43.31029, 34.471456)
  line L20 (43.31029, 34.471456) -> (34.471456, 43.31029)
  line L21 (34.471456, 43.31029) -> (15, 23.838835)
  line L22 (15, 23.838835) -> (15, 27.909903)
  arc A5 (12, 30.909903) -> (15, 27.909903) centre (15, 30.909903) ccw
  line L23 (12, 30.909903) -> (12, 31)
  arc A6 (12, 31) -> (9, 34) centre (9, 31) ccw
  line L24 (9, 34) -> (-9, 34)
  arc A7 (-9, 34) -> (-12, 31) centre (-9, 31) ccw
  line L25 (-12, 31) -> (-12, 30.909903)
  arc A8 (-15, 27.909903) -> (-12, 30.909903) centre (-15, 30.909903) ccw
  line L26 (-15, 27.909903) -> (-15, 23.838835)
  line L27 (-15, 23.838835) -> (-34.471456, 43.31029)
  line L28 (-34.471456, 43.31029) -> (-43.31029, 34.471456)
  line L29 (-43.31029, 34.471456) -> (-22.253048, 13.414214)
  circle A9 centre (10, 10) radius 0.9
  circle A10 centre (-10, -10) radius 0.9
  circle A11 centre (10, -10) radius 0.9
  circle A12 centre (-10, 10) radius 0.9
  line L30 (38.890873, -38.890873) -> (36.769553, -36.769553)
  circle A13 centre (36.769553, -36.769553) radius 0.95
  circle A14 centre (36.769553, 36.769553) radius 0.95
  circle A15 centre (-36.769553, 36.769553) radius 0.95
  circle A16 centre (-36.769553, -36.769553) radius 0.95
  line L31 (0, -34) -> (0, -31)
  circle A17 centre (0, -31) radius 0.95
  line L32 (0, 34) -> (0, 31)
  circle A18 centre (0, 31) radius 0.95
  circle A19 centre (0, 0) radius 0.95
  arc A20 (13.788582, 2.12132) -> (13.788582, -2.12132) centre (15.909903, 0) ccw
  dimension "d170" = 3
  dimension "d171" = 1.9
  dimension "d173" = 360
  dimension "d174" = 3
  dimension "d175" = 1.9
  dimension "d176" = 3
  dimension "d177" = 1.9
  dimension "d178" = 1.9
  constraint perpendicular L13 L30
  constraint midpoint L9 L31.start
  constraint perpendicular L9 L31
  constraint coincident L31.end A17.centre
  constraint midpoint L24 L32.start
  constraint perpendicular L24 L32
  constraint coincident L32.end A18.centre
  constraint coincident A19.centre origin
  measures "d171" diameter of A13
  measures "d174" distance of L31.start L31.end
  measures "d175" diameter of A17
  measures "d176" distance of L32.start L32.end
  measures "d177" diameter of A18
  measures "d178" diameter of A19
extrude "押し出し31" cut sketch "スケッチ31" against normal blind 2 contours A13 | A14 | A15 | A16 | A17 | A18 | A19 picked at (37.03376, -36.580044) picked at (36.611219, 37.043794) picked at (-36.927886, 37.043794) picked at (-36.927886, -36.495311) picked at (0.229907, -31.317035) picked at (-0.08819, 30.808025) picked at (0.579958, -0.294777)
sketch "スケッチ33" plane through (0, 0, 12) normal (0, 0, 1) x (-1, 0, 0)
  arc A0 (17.335447, 29.002709) -> (22.497291, 34.164553) centre (17.5, 34) ccw
  line L0 (17.335447, 29.002709) -> (17.12132, 28.788582)
  arc A1 (15, 27.909903) -> (17.12132, 28.788582) centre (15, 30.909903) ccw
  line L1 (15, 27.909903) -> (15, 23.838835)
  line L2 (15, 23.838835) -> (34.471456, 43.31029)
  line L3 (34.471456, 43.31029) -> (43.31029, 34.471456)
  line L4 (43.31029, 34.471456) -> (22.253048, 13.414214)
  line L5 (22.253048, 13.414214) -> (22.253048, -13.414214)
  line L6 (22.253048, -13.414214) -> (43.31029, -34.471456)
  line L7 (43.31029, -34.471456) -> (34.471456, -43.31029)
  line L8 (34.471456, -43.31029) -> (15, -23.838835)
  line L9 (15, -23.838835) -> (15, -27.909903)
  arc A2 (17.12132, -28.788582) -> (15, -27.909903) centre (15, -30.909903) ccw
  line L10 (17.12132, -28.788582) -> (17.335447, -29.002709)
  arc A3 (22.497291, -34.164553) -> (17.335447, -29.002709) centre (17.5, -34) ccw
  line L11 (22.497291, -34.164553) -> (34.471456, -46.138717)
  line L12 (34.471456, -46.138717) -> (46.138717, -34.471456)
  line L13 (46.138717, -34.471456) -> (23.667262, -12)
  line L14 (23.667262, -12) -> (23.667262, 12)
  line L15 (23.667262, 12) -> (46.138717, 34.471456)
  line L16 (46.138717, 34.471456) -> (34.471456, 46.138717)
  line L17 (34.471456, 46.138717) -> (22.497291, 34.164553)
  line L18 (15, -27.909903) -> (19.071068, -27.909903)
  arc A4 (-17.335447, -29.002709) -> (-22.497291, -34.164553) centre (-17.5, -34) ccw
  line L19 (-17.335447, -29.002709) -> (-17.12132, -28.788582)
  arc A5 (-15, -27.909903) -> (-17.12132, -28.788582) centre (-15, -30.909903) ccw
  line L20 (-15, -27.909903) -> (-15, -23.838835)
  line L21 (-15, -23.838835) -> (-34.471456, -43.31029)
  line L22 (-34.471456, -43.31029) -> (-43.31029, -34.471456)
  line L23 (-43.31029, -34.471456) -> (-22.253048, -13.414214)
  line L24 (-22.253048, -13.414214) -> (-22.253048, 13.414214)
  line L25 (-22.253048, 13.414214) -> (-43.31029, 34.471456)
  line L26 (-43.31029, 34.471456) -> (-34.471456, 43.31029)
  line L27 (-34.471456, 43.31029) -> (-15, 23.838835)
  line L28 (-15, 23.838835) -> (-15, 27.909903)
  arc A6 (-17.12132, 28.788582) -> (-15, 27.909903) centre (-15, 30.909903) ccw
  line L29 (-17.12132, 28.788582) -> (-17.335447, 29.002709)
  arc A7 (-22.497291, 34.164553) -> (-17.335447, 29.002709) centre (-17.5, 34) ccw
  line L30 (-22.497291, 34.164553) -> (-34.471456, 46.138717)
  line L31 (-34.471456, 46.138717) -> (-46.138717, 34.471456)
  line L32 (-46.138717, 34.471456) -> (-23.667262, 12)
  line L33 (-23.667262, 12) -> (-23.667262, -12)
  line L34 (-23.667262, -12) -> (-46.138717, -34.471456)
  line L35 (-46.138717, -34.471456) -> (-34.471456, -46.138717)
  line L36 (-34.471456, -46.138717) -> (-22.497291, -34.164553)
  line L37 (-15, -27.909903) -> (-19.071068, -27.909903)
  line L38 (-15, 27.909903) -> (-19.071068, 27.909903)
  line L39 (15, 27.909903) -> (19.071068, 27.909903)
  constraint tangent A2 L18
  constraint tangent A5 L37
  constraint tangent A6 L38
  constraint tangent A1 L39
extrude "押し出し32" add sketch "スケッチ33" along normal blind 7 contours L1 L2 L39 | L8 L9 L18 | L20 L21 L37 | L27 L28 L38 picked at (16.357023, 26.55288) picked at (16.357023, -26.55288) picked at (-16.357023, -26.55288) picked at (-16.357023, 26.55288)
sketch "スケッチ34" plane through (15, 0, 0) normal (-1, 0, 0) x (0, -1, 0)
  line L0 (23.838835, 19) -> (23.838835, 2)
  line L1 (23.838835, 2) -> (27.909903, 2)
  line L2 (27.909903, 2) -> (27.909903, 12)
  line L3 (27.909903, 12) -> (27.909903, 19)
  line L4 (27.909903, 19) -> (23.838835, 19)
  line L5 (23.838835, 19) -> (27.909903, 19)
  line L6 (27.909903, 19) -> (27.909903, 17)
  line L7 (27.909903, 17) -> (23.838835, 17)
  line L8 (23.838835, 17) -> (23.838835, 19)
  dimension "d183" = 4.071068
  dimension "d184" = 2
  constraint horizontal L5
  constraint vertical L6
  constraint horizontal L7
  constraint vertical L8
extrude "押し出し33" add sketch "スケッチ34" along normal blind 30 contours L0 L3 L4 L5 L6 L7 L8 picked at (25.195857, 18.333333)
mirror "ミラー2" about plane through (0, 0, 0) normal (0, 1, 0) of "押し出し33"
sketch "スケッチ35" plane through (0, 0, 17) normal (0, 0, 1) x (-1, 0, 0)
  line L0 (-19.62132, 36.12132) -> (-21.035534, 37.535534)
  arc A0 (-21.035534, 37.535534) -> (-13.964466, 37.535534) centre (-17.5, 34) ccw
  line L1 (-13.964466, 37.535534) -> (-15.37868, 36.12132)
  arc A1 (-19.62132, 36.12132) -> (-15.37868, 36.12132) centre (-17.5, 34) ccw
  line L2 (-19.071068, 27.909903) -> (-15, 27.909903)
  arc A2 (-17.12132, 28.788582) -> (-15, 27.909903) centre (-15, 30.909903) ccw
  line L3 (-17.12132, 28.788582) -> (-17.335447, 29.002709)
  arc A3 (-22.497291, 34.164553) -> (-17.335447, 29.002709) centre (-17.5, 34) ccw
  line L4 (-22.497291, 34.164553) -> (-34.471456, 46.138717)
  line L5 (-34.471456, 46.138717) -> (-46.138717, 34.471456)
  line L6 (-46.138717, 34.471456) -> (-23.667262, 12)
  line L7 (-23.667262, 12) -> (-23.667262, -12)
  line L8 (-23.667262, -12) -> (-46.138717, -34.471456)
  line L9 (-46.138717, -34.471456) -> (-34.471456, -46.138717)
  line L10 (-34.471456, -46.138717) -> (-22.497291, -34.164553)
  arc A4 (-17.335447, -29.002709) -> (-22.497291, -34.164553) centre (-17.5, -34) ccw
  line L11 (-17.335447, -29.002709) -> (-17.12132, -28.788582)
  arc A5 (-15, -27.909903) -> (-17.12132, -28.788582) centre (-15, -30.909903) ccw
  line L12 (-15, -27.909903) -> (-19.071068, -27.909903)
  line L13 (-19.071068, -27.909903) -> (-34.471456, -43.31029)
  line L14 (-34.471456, -43.31029) -> (-43.31029, -34.471456)
  line L15 (-43.31029, -34.471456) -> (-22.253048, -13.414214)
  line L16 (-22.253048, -13.414214) -> (-22.253048, 13.414214)
  line L17 (-22.253048, 13.414214) -> (-43.31029, 34.471456)
  line L18 (-43.31029, 34.471456) -> (-34.471456, 43.31029)
  line L19 (-34.471456, 43.31029) -> (-19.071068, 27.909903)
  line L20 (-22.497291, 34.164553) -> (-23.911505, 32.75034)
  line L21 (15, 27.909903) -> (19.071068, 27.909903)
  line L22 (19.071068, 27.909903) -> (34.471456, 43.31029)
  line L23 (34.471456, 43.31029) -> (43.31029, 34.471456)
  line L24 (43.31029, 34.471456) -> (22.253048, 13.414214)
  line L25 (22.253048, 13.414214) -> (22.253048, -13.414214)
  line L26 (22.253048, -13.414214) -> (43.31029, -34.471456)
  line L27 (43.31029, -34.471456) -> (34.471456, -43.31029)
  line L28 (34.471456, -43.31029) -> (19.071068, -27.909903)
  line L29 (19.071068, -27.909903) -> (15, -27.909903)
  arc A6 (17.12132, -28.788582) -> (15, -27.909903) centre (15, -30.909903) ccw
  line L30 (17.12132, -28.788582) -> (17.335447, -29.002709)
  arc A7 (22.497291, -34.164553) -> (17.335447, -29.002709) centre (17.5, -34) ccw
  line L31 (22.497291, -34.164553) -> (34.471456, -46.138717)
  line L32 (34.471456, -46.138717) -> (46.138717, -34.471456)
  line L33 (46.138717, -34.471456) -> (23.667262, -12)
  line L34 (23.667262, -12) -> (23.667262, 12)
  line L35 (23.667262, 12) -> (46.138717, 34.471456)
  line L36 (46.138717, 34.471456) -> (34.471456, 46.138717)
  line L37 (34.471456, 46.138717) -> (22.497291, 34.164553)
  arc A8 (17.335447, 29.002709) -> (22.497291, 34.164553) centre (17.5, 34) ccw
  line L38 (17.335447, 29.002709) -> (17.12132, 28.788582)
  arc A9 (15, 27.909903) -> (17.12132, 28.788582) centre (15, 30.909903) ccw
  line L39 (22.497291, 34.164553) -> (23.911505, 32.75034)
  line L40 (-22.497291, -34.164553) -> (-23.911505, -32.75034)
  line L41 (22.497291, -34.164553) -> (23.911505, -32.75034)
  constraint perpendicular L19 L20
  constraint perpendicular L22 L39
  constraint perpendicular L13 L40
  constraint perpendicular L28 L41
extrude "押し出し34" add sketch "スケッチ35" against normal blind 5 contours A0 L2 A2 L3 A3 L19 L20 | A4 L11 A5 L12 L13 L40 | L21 L22 A8 L38 A9 L39 | L28 L29 A6 L30 A7 L41 picked at (-22.901299, 32.954809) picked at (-22.901299, -32.954809) picked at (22.901299, 32.954809) picked at (22.901299, -32.954809)
sketch "スケッチ36" plane through (0, 0, 19) normal (0, 0, 1) x (-1, 0, 0)
  line L0 (15, -27.909903) -> (19.071068, -27.909903)
  line L1 (19.071068, -27.909903) -> (15, -23.838835)
  line L2 (15, -23.838835) -> (-15, -23.838835)
  line L3 (-15, -23.838835) -> (-19.071068, -27.909903)
  line L4 (-19.071068, -27.909903) -> (-15, -27.909903)
  line L5 (-15, -27.909903) -> (15, -27.909903)
  line L6 (-15, 27.909903) -> (-19.071068, 27.909903)
  line L7 (-19.071068, 27.909903) -> (-15, 23.838835)
  line L8 (-15, 23.838835) -> (15, 23.838835)
  line L9 (15, 23.838835) -> (19.071068, 27.909903)
  line L10 (19.071068, 27.909903) -> (15, 27.909903)
  line L11 (15, 27.909903) -> (-15, 27.909903)
  line L12 (15, -23.838835) -> (12, -23.838835)
  line L13 (12, -23.838835) -> (12, 23.838835)
  line L14 (12, 23.838835) -> (15, 23.838835)
  line L15 (15, 23.838835) -> (15, -23.838835)
  line L16 (-15, -23.838835) -> (-12, -23.838835)
  line L17 (-12, -23.838835) -> (-12, 23.838835)
  line L18 (-12, 23.838835) -> (-15, 23.838835)
  line L19 (-15, 23.838835) -> (-15, -23.838835)
  line L20 (15, 23.838835) -> (-15, -23.838835)
  line L21 (-15, -23.838835) -> (-16.269581, -23.039983)
  line L22 (-16.269581, -23.039983) -> (-13.73042, -24.637687)
  line L23 (-13.73042, -24.637687) -> (16.269581, 23.039983)
  line L24 (16.269581, 23.039983) -> (13.73042, 24.637687)
  line L25 (13.73042, 24.637687) -> (-16.269581, -23.039983)
  line L26 (-1.75, 0) -> (-22.5, 0)
  line L27 (13.73042, -24.637687) -> (-16.269581, 23.039983)
  line L28 (-13.73042, 24.637687) -> (16.269581, -23.039983)
  dimension "d191" = 3
  dimension "d192" = 3
  dimension "d193" = 1.5
  dimension "d194" = 3
  constraint horizontal L12
  constraint vertical L13
  constraint horizontal L14
  constraint vertical L15
  constraint horizontal L16
  constraint vertical L17
  constraint horizontal L18
  constraint vertical L19
  constraint perpendicular L20 L21
  constraint perpendicular L22 L23
  constraint parallel L22 L24
  constraint parallel L23 L25
  constraint perpendicular L20 L22
extrude "押し出し35" add sketch "スケッチ36" against normal blind 2 contours L2 L12 L13 L15 L27 L28 | L2 L12 L13 L27 | L13 L15 L23 L28 | L2 L16 L17 L20 L23 | L17 L19 L20 L25 | L13 L23 L27 L28 | L13 L15 L20 L23 | L2 L16 L17 L23 | L17 L19 L25 L26 | L17 L20 L23 L27 | L17 L20 L25 L27 | L20 L23 L27 L28 | L8 L13 L14 L20 L25 | L13 L20 L23 L28 | L17 L19 L26 L27 | L20 L25 L27 L28 | L8 L13 L14 L25 | L13 L20 L25 L28 | L8 L17 L18 L19 L27 L28 | L17 L25 L27 L28 | L8 L17 L18 L28 picked at (13, -19.721477) picked at (12.409254, -23.188426) picked at (14, -5.418176) picked at (-13, -21.59917) picked at (-13, -18.78263) picked at (8, -13.652892) picked at (13, 18.78263) picked at (-12.409254, -23.188426) picked at (-14, -12.425607) picked at (-8, -14.591739) picked at (-8.295373, -12.244622) picked at (0.295373, -1.40827) picked at (13, 21.59917) picked at (8.295373, 12.244622) picked at (-14, 12.425607) picked at (-0.295373, 1.40827) picked at (12.409254, 23.188426) picked at (8, 14.591739) picked at (-13, 19.721477) picked at (-8, 13.652892) picked at (-12.409254, 23.188426)
